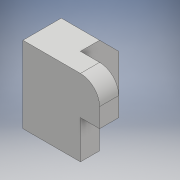
# Autodesk Inventor part: 47
Saved by Autodesk Inventor 2017 (Build 210142000, 142)
## iProperties
Part Number: 47
Material: 一般
Document SubType Name: Modeling
Designer: Brian
Density: 1 g/cm^3
Appearance: 預設
Author: Brian
Autodesk Inventor part; units mm, degrees
ref_plane "YZ Plane" through (0, 0, 0) normal (1, 0, 0) x (0, 1, 0)
ref_plane "XZ Plane" through (0, 0, 0) normal (0, 1, 0) x (-1, 0, 0)
ref_plane "XY Plane" through (0, 0, 0) normal (0, 0, 1) x (1, 0, 0)
sketch "草圖1" plane through (0, 0, 0) normal (0, 1, 0) x (-1, 0, 0)
  line L0 (0, 0) -> (-30, 0)
  line L1 (-30, 0) -> (-30, -40)
  line L2 (-30, -40) -> (0, -40)
  line L3 (0, -40) -> (0, 0)
  line L4 (-30, 0) -> (-40, 0)
  line L5 (-40, 0) -> (-40, -20)
  line L6 (-40, -20) -> (-30, -20)
  line L7 (-30, -20) -> (-30, 0)
  dimension "d0" = 30
  dimension "d1" = 40
  dimension "d2" = 10
  dimension "d3" = 20
  constraints: 16 end point, 4 parallel, 2 horizontal, 2 perpendicular
  measures "d0" distance of L1.end L2.end
  measures "d1" distance of L0.end L1.end
  measures "d2" distance of L5.end L6.end
  measures "d3" distance of L4.end L5.end
extrude "擠出1" add sketch "草圖1" along normal blind 10
sketch "草圖2" plane through (0, 10, 0) normal (0, 1, 0) x (1, 0, 0)
  line L0 (0, 0) -> (40, 0) projected
  line L1 (30, 40) -> (0, 40) projected
  line L2 (0, 0) -> (20, 0)
  line L3 (20, 0) -> (20, 40)
  line L4 (20, 40) -> (0, 40)
  line L5 (0, 40) -> (0, 0)
  dimension "d6" = 20
  constraints: 8 end point, 2 parallel, 1 horizontal, 1 perpendicular, 1 point on line
  measures "d6" distance between parallel lines of L5 L3
extrude "擠出2" add sketch "草圖2" along normal blind 20
chamfer "倒角1" distance 10 angle 45 1 edges at (10, 30, 0)
fillet "圓角1" radius 10 1 edges at (40, 5, 0)
